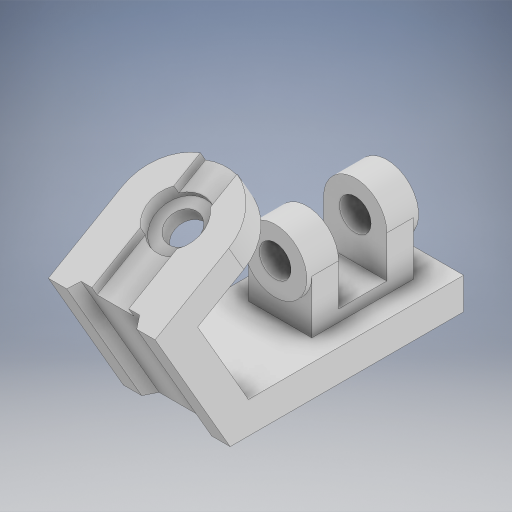
# Autodesk Inventor part: 1.1
Saved by Autodesk Inventor 2024 (Build 280153000, 153)
## iProperties
Created: 2024-01-18
Part Number: 1.1
Material: Generic
Document SubType Name: Modeling
Designer: Alex
Density: 1 g/cm^3
Appearance: Default
Author: Alex
Autodesk Inventor part; units mm, degrees
ref_plane "YZ Plane" through (0, 0, 0) normal (1, 0, 0) x (0, 1, 0)
sketch "Sketch1" plane through (0, 0, 0) normal (0, 1, 0) x (-1, 0, 0)
  line L0 (0, 0) -> (-64, 0)
  line L1 (-64, 0) -> (-64, 140)
  line L2 (-64, 140) -> (0, 140)
  line L3 (0, 140) -> (0, 0)
  dimension "d0" = 140
  dimension "d1" = 64
  constraints: 8 end point, 2 parallel, 1 horizontal, 1 perpendicular
  measures "d0" distance of L0.end L1.end
  measures "d1" distance of L1.end L2.end
extrude "Extrusion1" add sketch "Sketch1" along normal blind 19
sketch "Sketch3" plane through (64, 0, 140) normal (1, 0, 0) x (0, 0, -1)
  line L0 (0, 0) -> (-36, 62.3538)
  line L1 (0, 0) -> (72, 0) construction
  line L2 (-36, 62.3538) -> (-19.5455, 71.8538)
  line L3 (-19.5455, 71.8538) -> (21.9393, 0)
  line L4 (0, 0) -> (140, 0) projected
  line L5 (21.9393, 0) -> (0, 0)
  dimension "d4" = 72
  dimension "d5" = 120
  dimension "d6" = 19
  dimension "d7" = 90
  constraints: 10 end point, 1 collinear, 1 equal length, 1 horizontal, 1 parallel, 1 point on line
  measures "d4" distance of L0.start L0.end
  measures "d5" angle of L1 L0
  measures "d6" distance of L0.end L2.end
  measures "d7" angle of L2 L3
extrude "Extrusion2" add sketch "Sketch3" against normal up to surface (64 mm away)
sketch "Sketch4" plane through (0, 62.3538, 176) normal (0, 0.8660254, 0.5) x (1, 0, 0)
  line L0 (64, 0) -> (0, 0) construction
  line L1 (32, 0) -> (32, 51) construction
  line L2 (32, 0) -> (83, 0) construction
  arc A0 (64, 51) -> (0, 51) centre (32, 51) ccw
  line L3 (0, 51) -> (0, 0)
  line L4 (64, 51) -> (64, 0)
  line L5 (0, 0) -> (64, 0)
  point P0 (0, 121.2436)
  dimension "d10" = 51
  dimension "d11" = 90
  dimension "d12" = 64
  constraints: 10 end point, 2 point on circle, 2 tangent, 1 centre point, 1 coincident, 1 collinear, 1 horizontal, 1 midpoint, 1 perpendicular, 1 vertical
  measures "d10" distance of L1.start L1.end
  measures "d11" angle of L2 L1
  measures "d12" diameter of A0
extrude "Extrusion3" add sketch "Sketch4" along normal blind 18
sketch "Sketch5" plane through (0, 77.9423, 185) normal (0, 0.8660254, 0.5) x (1, 0, 0)
  line L0 (0, 0) -> (64, 0) construction
  line L1 (32, 0) -> (32, 51) construction
  circle A0 centre (32, 51) radius 9.5
  point P0 (0, 121.2436)
  dimension "d15" = 51
  dimension "d16" = 19
  constraints: 2 end point, 1 centre point, 1 coincident, 1 midpoint, 1 vertical
  measures "d15" distance of L1.start L1.end
  measures "d16" diameter of A0
extrude "Extrusion4" cut sketch "Sketch5" against normal up to surface (18 mm away)
sketch "Sketch6" plane through (0, 77.9423, 185) normal (0, 0.8660254, 0.5) x (1, 0, 0)
  circle A0 centre (32, 51) radius 9.5 construction
  circle A1 centre (32, 51) radius 16
  point P0 (0, 121.2436)
  dimension "d19" = 32
  constraints: 1 centre point, 1 coincident
  measures "d19" diameter of A1
extrude "Extrusion5" cut sketch "Sketch6" against normal blind 9
sketch "Sketch9" plane through (0, 77.9423, 185) normal (0, 0.8660254, 0.5) x (1, 0, 0)
  line L0 (0, 0) -> (64, 0) construction
  line L1 (32, 0) -> (32, 83) construction
  arc A0 (64, 51) -> (0, 51) centre (32, 51) ccw construction
  line L2 (32, 0) -> (115, 0) construction
  arc A1 (64, 51) -> (0, 51) centre (32, 51) ccw construction
  line L3 (32, 83) -> (43, 83) construction
  line L4 (32, 83) -> (43, 83) construction
  line L5 (43, 83) -> (21, 83)
  line L6 (21, 83) -> (21, 0)
  line L7 (21, 0) -> (43, 0)
  line L8 (43, 0) -> (43, 83)
  point P0 (0, 121.2436)
  dimension "d22" = 90
  dimension "d23" = 11
  dimension "d24" = 0
  dimension "d25" = 22
  dimension "d26" = 83
  constraints: 16 end point, 3 horizontal, 2 equal length, 2 parallel, 1 midpoint, 1 perpendicular, 1 point on circle, 1 tangent
  measures "d22" angle of L2 L1
  measures "d23" distance of L1.end L3.end
  measures "d24" distance between parallel lines of L3 L4
  measures "d25" distance of L7.end L6.end
  measures "d26" distance of L6.end L5.end
extrude "Extrusion6" cut sketch "Sketch9" against normal blind 6
ref_plane "Work Plane1" through (64, 103.4423, 140.8327) normal (0, 0.8660254, 0.5) x (1, 0, 0)
sketch "Sketch10" plane through (64, 103.4423, 140.8327) normal (0, 0.8660254, 0.5) x (1, 0, 0)
  line L0 (-64, -51) -> (-43, -51) construction
  line L1 (-64, -51) -> (-64, -45) construction
  line L2 (-64, 0) -> (-64, -51) construction
  line L3 (-64, -45) -> (0, -45) construction
  line L4 (0, -51) -> (0, 0) construction
  line L5 (-32, -45) -> (-32, -51) construction
  line L6 (-21, -51) -> (-43, -51) construction
  line L7 (-32, -51) -> (-11, -51) construction
  line L8 (-32, -51) -> (-11, -51) construction
  line L9 (-11, -51) -> (-53, -51)
  line L10 (-11, -51) -> (31, -51) construction
  line L11 (-53, -51) -> (-49.5359, -45)
  line L12 (-53, -51) -> (-46.0718, -51) construction
  line L13 (-11, -51) -> (-14.4641, -45)
  line L14 (-49.5359, -45) -> (-14.4641, -45)
  point P0 (-64, 70.2436)
  dimension "d29" = 6
  dimension "d30" = 21
  dimension "d31" = 0
  dimension "d32" = 42
  dimension "d33" = 180
  dimension "d34" = 60
  constraints: 22 end point, 5 horizontal, 3 equal length, 3 point on line, 2 collinear, 2 midpoint, 1 symmetric about line
  measures "d29" distance of L0.start L1.end
  measures "d30" distance of L5.end L7.end
  measures "d31" distance between parallel lines of L7 L8
  measures "d32" distance of L8.end L9.end
  measures "d33" angle of L10 L9
  measures "d34" angle of L12 L11
extrude "Extrusion7" cut sketch "Sketch10" against normal up to surface surface through (32, 0, 70) normal (0, 1, 0)
sketch "Sketch11" plane through (0, 19, 0) normal (0, 1, 0) x (1, 0, 0)
  line L0 (64, 0) -> (0, 0) construction
  line L1 (0, 0) -> (0, -140) construction
  line L2 (64, 0) -> (0, 0) construction
  line L3 (0, 0) -> (0, -17) construction
  line L4 (0, -17) -> (64, -17) construction
  line L5 (64, -17) -> (64, 0) construction
  line L6 (64, 0) -> (51, 0) construction
  line L7 (51, 0) -> (51, -17) construction
  line L8 (51, -17) -> (64, -17) construction
  line L9 (64, -17) -> (64, 0) construction
  line L10 (51, -17) -> (13, -17)
  line L11 (13, -17) -> (13, -78)
  line L12 (13, -78) -> (51, -78)
  line L13 (51, -78) -> (51, -17)
  dimension "d39" = 17
  dimension "d40" = 13
  dimension "d41" = 17
  dimension "d42" = 38
  dimension "d43" = 61
  constraints: 24 end point, 6 parallel, 3 horizontal, 3 perpendicular, 1 point on line
  measures "d39" distance of L3.end L2.end
  measures "d40" distance of L8.end L7.end
  measures "d41" distance of L7.end L6.end
  measures "d42" distance of L12.end L11.end
  measures "d43" distance of L11.end L10.end
extrude "Extrusion8" add sketch "Sketch11" along normal blind 7
sketch "Sketch12" plane through (0, 26, 0) normal (0, 1, 0) x (1, 0, 0)
  line L0 (13, -78) -> (13, -17) construction
  line L1 (13, -47.5) -> (51, -47.5) construction
  line L2 (51, -17) -> (51, -78) construction
  line L3 (13, -17) -> (51, -17) construction
  line L4 (32, -17) -> (32, -78) construction
  line L5 (13, -62) -> (51, -62) construction
  line L6 (51, -62) -> (51, -33) construction
  line L7 (51, -33) -> (13, -33) construction
  line L8 (13, -33) -> (13, -62) construction
  line L9 (13, -62) -> (51, -33) construction
  line L10 (51, -62) -> (13, -33) construction
  line L11 (13, -17) -> (51, -17)
  line L12 (51, -17) -> (51, -33)
  line L13 (51, -33) -> (13, -33)
  line L14 (13, -33) -> (13, -17)
  line L15 (51, -78) -> (13, -78) projected
  line L16 (13, -62) -> (51, -62)
  line L17 (51, -62) -> (51, -78)
  line L18 (51, -78) -> (13, -78)
  line L19 (13, -78) -> (13, -62)
  point P0 (0, 0)
  point P1 (32, -47.5)
  dimension "d46" = 29
  dimension "d47" = 45
  dimension "d48" = 45
  constraints: 32 end point, 6 midpoint, 6 parallel, 3 horizontal, 3 perpendicular, 2 point on line, 1 vertical
  measures "d46" distance of L6.end L5.end
  measures "d47" distance between parallel lines of L15 L7
  measures "d48" distance between parallel lines of L13 L15
extrude "Extrusion9" add sketch "Sketch12" along normal blind 25 contours L11 L12 L13 L14
ref_plane "Work Plane2" through (32, 26, 47.5) normal (0, 0, 1) x (1, 0, 0)
sketch "Sketch14" plane through (51, 19, 17) normal (0, 0, -1) x (-1, 0, 0)
  line L0 (0, 32) -> (38, 32) projected
  arc A0 (38, 32) -> (0, 32) centre (19, 32) ccw
  point P0 (51, -19)
  constraints: 2 end point, 2 point on circle, 1 centre point, 1 midpoint
extrude "Extrusion10" add sketch "Sketch14" against normal up to surface (16 mm away)
sketch "Sketch15" plane through (51, 19, 17) normal (0, 0, -1) x (-1, 0, 0)
  arc A0 (38, 32) -> (0, 32) centre (19, 32) ccw construction
  line L0 (38, 0) -> (38, 32) construction
  circle A1 centre (19, 32) radius 19
  point P0 (51, -19)
  constraints: 1 coincident, 1 horizontal alignment, 2 other
extrude "Extrusion11" add sketch "Sketch15" along normal blind 3
sketch "Sketch16" plane through (32, 51, 14) normal (0, 0, -1) x (-1, 0, 0)
  circle A0 centre (0, 0) radius 9.5
  point P0 (32, -51)
  dimension "d55" = 19
  constraints: 1 centre point
  measures "d55" diameter of A0
extrude "Extrusion12" cut sketch "Sketch16" against normal up to surface (19 mm away)
mirror "Mirror1" about plane through (32, 26, 47.5) normal (0, 0, 1) of "Extrusion10", "Extrusion11", "Extrusion12", "Extrusion9"
body "Solid1"
